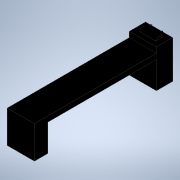
# Autodesk Inventor part: carSpacer
Saved by Autodesk Inventor 2020 (Build 240168000, 168)
## iProperties
Created: 2019-08-05
Part Number: carSpacer
Material: Generic
Document SubType Name: Modeling
Designer: n10208577
Density: 1 g/cm^3
Appearance: Default
Author: n10208577
Autodesk Inventor part; units mm, degrees
ref_plane "YZ Plane" through (0, 0, 0) normal (1, 0, 0) x (0, 1, 0)
ref_plane "XZ Plane" through (0, 0, 0) normal (0, 1, 0) x (-1, 0, 0)
ref_plane "XY Plane" through (0, 0, 0) normal (0, 0, 1) x (1, 0, 0)
sketch "Sketch1" plane through (0, 0, 0) normal (0, 1, 0) x (-1, 0, 0)
  line L0 (0, 0) -> (10, 0)
  circle A0 centre (10, 0) radius 1.5
  line L1 (0, 0) -> (-10, 0)
  circle A1 centre (-10, 0) radius 1.5
  line L2 (0, 0) -> (0, 6)
  line L3 (0, 6) -> (15, 6)
  line L4 (15, 6) -> (15, 16)
  line L5 (15, 16) -> (-15, 16)
  line L6 (-15, 16) -> (-15, 6)
  line L7 (-15, 6) -> (0, 6)
  dimension "d0" = 10
  dimension "d1" = 3
  dimension "d2" = 10
  dimension "d3" = 3
  dimension "d4" = 6
  dimension "d5" = 15
  dimension "d7" = 10
  dimension "d8" = 30
  dimension "d9" = 10
  constraints: 16 end point, 3 perpendicular, 2 centre point, 2 coincident, 2 horizontal, 2 vertical
  measures "d0" distance of L0.start L0.end
  measures "d1" diameter of A0
  measures "d2" distance of L0.start L1.end
  measures "d3" diameter of A1
  measures "d4" distance of L0.start L2.end
  measures "d5" distance of L2.end L3.end
  measures "d7" distance of L3.end L4.end
  measures "d8" distance of L4.end L5.end
  measures "d9" distance of L5.end L6.end
extrude "Extrusion1" add sketch "Sketch1" along normal blind 5
fillet "Fillet1" radius 5 2 edges at (0, 5, 6) (0, 5, 16)
sketch "Sketch2" plane through (0, 0, 0) normal (0, -1, 0) x (1, 0, 0)
  line L0 (0, 0) -> (0, -5)
  line L1 (0, -5) -> (-25, -5)
  line L2 (-25, -5) -> (-25, 25)
  line L3 (-25, 25) -> (25, 25)
  line L4 (25, 25) -> (25, -5)
  line L5 (25, -5) -> (0, -5)
  dimension "d13" = 5
  dimension "d14" = 25
  dimension "d15" = 30
  dimension "d16" = 50
  dimension "d17" = 30
  constraints: 12 end point, 3 perpendicular, 2 vertical
  measures "d13" distance of L0.start L0.end
  measures "d14" distance of L0.end L1.end
  measures "d15" distance of L1.end L2.end
  measures "d16" distance of L2.end L3.end
  measures "d17" distance of L3.end L4.end
extrude "Extrusion2" add sketch "Sketch2" along normal blind 70
sketch "Sketch3" plane through (-25, 0, 25) normal (0, 0, 1) x (1, 0, 0)
  line L0 (0, 0) -> (0, -70) projected
  line L1 (0, 0) -> (0, -20)
  line L2 (0, -20) -> (50, -20)
  line L3 (50, 0) -> (50, -70) projected
  line L4 (50, -20) -> (50, -10)
  line L5 (50, -10) -> (0, -10)
  point P0 (25, 0)
  dimension "d20" = 20
  dimension "d21" = 10
  constraints: 8 end point, 2 perpendicular, 2 point on line, 1 midpoint
  measures "d20" distance of L0.start L1.end
  measures "d21" distance of L2.end L4.end
extrude "Extrusion3" add sketch "Sketch3" along normal blind 225
sketch "Sketch4" plane through (-25, -20, 25) normal (0, -1, 0) x (1, 0, 0)
  line L0 (50, 0) -> (50, 225) projected
  line L1 (50, 225) -> (50, 200)
  line L2 (50, 200) -> (0, 200)
  line L3 (0, 0) -> (0, 225) projected
  line L4 (0, 225) -> (0, 200)
  line L5 (0, 225) -> (50, 225)
  point P0 (25, -25)
  dimension "d24" = 25
  constraints: 8 end point, 3 perpendicular, 2 point on line
  measures "d24" distance of L0.end L1.end
extrude "Extrusion4" add sketch "Sketch4" along normal blind 50
body "Solid1"
